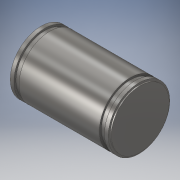
# Autodesk Inventor part: MiddleShaftCJE
Saved by Autodesk Inventor 2018 (Build 220112000, 112)
## iProperties
Created: 2018-01-21
Part Number: MiddleShaftCJE
Material: Steel, Alloy
Document SubType Name: Modeling
Designer: textboox5
Density: 7.73 g/cm^3
Appearance: Semi-Polished
Author: textboox5
Autodesk Inventor part; units mm, degrees
ref_plane "YZ Plane" through (0, 0, 0) normal (1, 0, 0) x (0, 1, 0)
ref_plane "XZ Plane" through (0, 0, 0) normal (0, 1, 0) x (-1, 0, 0)
ref_plane "XY Plane" through (0, 0, 0) normal (0, 0, 1) x (1, 0, 0)
sketch "Sketch1" plane through (0, 0, 0) normal (0, 0, 1) x (1, 0, 0)
  line L0 (1828.8, 1168.4) -> (1828.8, 1244.6)
  line L1 (1828.8, 1244.6) -> (1981.2, 1244.6)
  line L2 (1981.2, 1244.6) -> (1981.2, 1168.4)
  line L3 (1981.2, 1117.6) -> (-1981.2, 1117.6)
  line L4 (-1981.2, 1168.4) -> (-1981.2, 1244.6)
  line L5 (-1981.2, 1244.6) -> (-1828.8, 1244.6)
  line L6 (-1828.8, 1244.6) -> (-1828.8, 1168.4)
  line L7 (0, 0) -> (0, 1117.6) construction
  line L8 (-1981.2, 0) -> (1981.2, 0) construction
  line L9 (-1981.2, 1168.4) -> (-2032, 1168.4)
  line L10 (-2032, 1168.4) -> (-2032, 0)
  line L11 (-2032, 0) -> (-1981.2, 0)
  line L12 (-1981.2, 1117.6) -> (-1981.2, 0)
  line L13 (1981.2, 1168.4) -> (2032, 1168.4)
  line L14 (2032, 1168.4) -> (2032, 0)
  line L15 (2032, 0) -> (1981.2, 0)
  line L16 (1981.2, 0) -> (1981.2, 1117.6)
  line L17 (-1625.6, 1168.4) -> (-1625.6, 1244.6)
  line L18 (-1625.6, 1244.6) -> (1625.6, 1244.6)
  line L19 (1625.6, 1244.6) -> (1625.6, 1168.4)
  line L20 (-1828.8, 1168.4) -> (-1625.6, 1168.4)
  line L21 (1625.6, 1168.4) -> (1828.8, 1168.4)
  dimension "d1" = 2489.2
  dimension "d3" = 152.4
  dimension "d4" = 50.8
  dimension "d5" = 50.8
  dimension "d8" = 203.2
  dimension "d9" = 2336.8
  dimension "d10" = 3251.2
  constraints: 44 end point, 17 perpendicular, 4 horizontal, 2 collinear, 2 midpoint, 2 point on line, 2 vertical, 8 other
  measures "d1" diameter of L5 L8
  measures "d3" distance between parallel lines of L6 L4
  measures "d4" distance between parallel lines of L12 L10
  measures "d5" distance between parallel lines of L9 L3
  measures "d8" distance between parallel lines of L17 L6
  measures "d9" diameter of L20 L8
  measures "d10" distance between parallel lines of L19 L17
revolve "Revolution1" add sketch "Sketch1" angle 360 about axis through (-1981.2, 0, 0) along (1, 0, 0)
body "Solid1"
